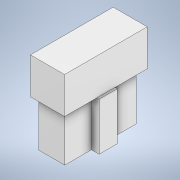
# Autodesk Inventor part: Connector_female
Saved by Autodesk Inventor 2020 (Build 240168000, 168)
## iProperties
Created: 2022-03-29
Part Number: Connector_female
Material: Tworzywo sztuczne ABS
Document SubType Name: Modeling
Designer: mikoma
Density: 1.06 g/cm^3
Appearance: Gładki — biały
Mass: 2.22923 g
Surface Area: 11.733 cm^2
Volume: 2.10304 cm^3
Author: mikoma
Autodesk Inventor part; units mm, degrees
ref_plane "YZ Plane" through (0, 0, 0) normal (1, 0, 0) x (0, 1, 0)
ref_plane "XZ Plane" through (0, 0, 0) normal (0, 1, 0) x (-1, 0, 0)
ref_plane "XY Plane" through (0, 0, 0) normal (0, 0, 1) x (1, 0, 0)
sketch "Szkic1" plane through (0, 0, 0) normal (0, 1, 0) x (-1, 0, 0)
  line L0 (-2.85, 7.85) -> (2.85, 7.85)
  line L1 (2.85, 7.85) -> (2.85, -7.85)
  line L2 (2.85, -7.85) -> (-2.85, -7.85)
  line L3 (-2.85, -7.85) -> (-2.85, 7.85)
  line L4 (-2.85, 7.85) -> (2.85, -7.85) construction
  line L5 (2.85, 7.85) -> (-2.85, -7.85) construction
  line L6 (-2.85, 2) -> (-4.55, 2)
  line L7 (-4.55, 2) -> (-4.55, -2)
  line L8 (-4.55, -2) -> (-2.85, -2)
  line L9 (-2.85, -2) -> (-2.85, 2)
  point P0 (0, 0)
  dimension "d0" = 15.7
  dimension "d1" = 5.7
  dimension "d2" = 4
  dimension "d3" = 7.4
  dimension "d4" = 2
  constraints: 20 end point, 4 parallel, 2 horizontal, 2 midpoint, 2 perpendicular, 1 point on line
  measures "d0" distance of L0.end L1.end
  measures "d1" distance of L1.end L2.end
  measures "d2" distance of L8.end L6.start
  measures "d3" distance between parallel lines of L1 L7
  measures "d4" distance from line of point (0, 0) L6
extrude "Wyciągnięcie proste1" add sketch "Szkic1" along normal blind 10.5
sketch "Szkic2" plane through (0, 10.5, 0) normal (0, 1, 0) x (1, 0, 0)
  line L0 (-3.45, -9.1) -> (4.05, -9.1)
  line L1 (4.05, -9.1) -> (4.05, 9.1)
  line L2 (4.05, 9.1) -> (-3.45, 9.1)
  line L3 (-3.45, 9.1) -> (-3.45, -9.1)
  line L4 (-3.45, -9.1) -> (4.05, 9.1) construction
  line L5 (4.05, -9.1) -> (-3.45, 9.1) construction
  line L6 (-2.85, 7.85) -> (-2.85, -7.85) projected
  line L7 (2.85, 2) -> (2.85, 7.85) projected
  point P0 (0, 0)
  point P1 (0.3, 0)
  point P2 (0.3, 0)
  dimension "d7" = 18.2
  dimension "d8" = 7.5
  dimension "d10" = 1.2
  constraints: 12 end point, 3 midpoint, 2 parallel, 1 horizontal, 1 horizontal alignment, 1 perpendicular
  measures "d7" distance of L2.end L0.start
  measures "d8" distance of L1.end L2.end
  measures "d10" distance between parallel lines of L7 L1
extrude "Wyciągnięcie proste2" add sketch "Szkic2" along normal blind 8
